HACKberry_R (Autodesk Fusion 360 archive; units mm, degrees)
design "SS12SDP2"
Autodesk Fusion 360 part; units mm, degrees
box "直方体プリミティブ1" add length 10.2 width 4 height 4.5 placed x (0, 0, 1) y (1, 0, 0) z (0, 1, 0) at (0, 0, 0) makes body 1
sketch "スケッチ2" plane through (0, 4.5, 0) normal (0, 1, 0) x (-1, 0, 0)
  line L0 (0, 10.2) -> (-4, 10.2)
  line L1 (-4, 10.2) -> (-4, 0)
  line L2 (-4, 0) -> (0, 0)
  line L3 (0, 0) -> (0, 10.2)
  line L4 (0, 0) -> (-4, 10.2) construction
  line L5 (0, 10.2) -> (-4, 0) construction
  line L6 (-2.6, 3.35) -> (-1.4, 3.35)
  line L7 (-1.4, 3.35) -> (-1.4, 6.85)
  line L8 (-1.4, 6.85) -> (-2.6, 6.85)
  line L9 (-2.6, 6.85) -> (-2.6, 3.35)
  line L10 (-2.6, 3.35) -> (-1.4, 6.85) construction
  line L11 (-1.4, 3.35) -> (-2.6, 6.85) construction
  point P0 (-2, 5.1)
  dimension "d6" = 1.2
  dimension "d7" = 3.5
  measures "d6" distance of L7.end L8.end
  measures "d7" distance of L6.end L7.end
extrude "押し出し1" cut sketch "スケッチ2" against normal blind 1 contours L6 L7 L8 L9 bodies 1
sketch "スケッチ3" plane through (0, 3.5, 0) normal (0, 1, 0) x (-1, 0, 0)
  line L0 (-2.6, 6.85) -> (-2.6, 3.35)
  line L1 (-2.6, 3.35) -> (-1.4, 3.35)
  line L2 (-1.4, 3.35) -> (-1.4, 6.85)
  line L3 (-1.4, 6.85) -> (-2.6, 6.85)
  line L4 (-1.4, 3.35) -> (-2.6, 3.35)
  line L5 (-2.6, 3.35) -> (-2.6, 5.1)
  line L6 (-2.6, 5.1) -> (-1.4, 5.1)
  line L7 (-1.4, 5.1) -> (-1.4, 3.35)
extrude "押し出し2" add sketch "スケッチ3" along normal blind 3 separate body contours L0 L1 L2 L4 L5 L6 L7 makes body 2
sketch "スケッチ4" plane through (0, 0, 0) normal (0, -1, 0) x (1, 0, 0)
  line L0 (4, 10.2) -> (0, 10.2)
  line L1 (0, 10.2) -> (0, 0)
  line L2 (0, 0) -> (4, 0)
  line L3 (4, 0) -> (4, 10.2)
  line L4 (2.2, 4.8) -> (1.8, 4.8)
  line L5 (1.8, 4.8) -> (1.8, 5.4)
  line L6 (1.8, 5.4) -> (2.2, 5.4)
  line L7 (2.2, 5.4) -> (2.2, 4.8)
  line L8 (2.2, 4.8) -> (1.8, 5.4) construction
  line L9 (1.8, 4.8) -> (2.2, 5.4) construction
  line L10 (1.4, 5.1) -> (2.6, 5.1)
  line L11 (1.8, 2.26) -> (1.8, 2.86)
  line L12 (2.2, 2.26) -> (1.8, 2.26)
  line L13 (1.8, 2.86) -> (2.2, 2.86)
  line L14 (2.2, 2.26) -> (1.8, 2.86) construction
  line L15 (1.8, 2.26) -> (2.2, 2.86) construction
  line L16 (2.2, 2.86) -> (2.2, 2.26)
  line L17 (1.8, 7.34) -> (1.8, 7.94)
  line L18 (2.2, 7.34) -> (1.8, 7.34)
  line L19 (1.8, 7.94) -> (2.2, 7.94)
  line L20 (2.2, 7.34) -> (1.8, 7.94) construction
  line L21 (1.8, 7.34) -> (2.2, 7.94) construction
  line L22 (2.2, 7.94) -> (2.2, 7.34)
  point P0 (2, 5.1)
  point P1 (2, 2.56)
  point P2 (2, 7.64)
  dimension "d12" = 0.4
  dimension "d13" = 0.6
  dimension "d16" = 0
  dimension "d17" = 2.54
  measures "d12" distance of L5.end L6.end
  measures "d13" distance of L4.end L5.end
extrude "押し出し3" add sketch "スケッチ4" along normal blind 3.4 separate body contours L4 L5 L7 L10 | L5 L6 L7 L10 | L11 L12 L13 L16 | L17 L18 L19 L22 makes body 3 at (1.8, -1.1333, 2.46) makes body 4 at (1.8, -1.1333, 7.54) makes body 5 at (2.2, -1.1333, 5.2)
chamfer "面取り1" distance 0.2 angle 45 8 edges at (2, 4.5, 10.2) (4, 2.25, 10.2) (4, 4.5, 5.1) (0, 4.5, 5.1) (0, 2.25, 10.2) (4, 2.25, 0) (2, 4.5, 0) (0, 2.25, 0) on bodies 1
sketch "スケッチ5" plane through (0, 0, 0) normal (-1, 0, 0) x (0, 0, 1)
  line L0 (0.2, 0) -> (10, 0)
  line L1 (0, 2.3446) -> (10.2, 2.3446)
  line L2 (10, 0) -> (10, 4.3)
  line L3 (10, 4.3) -> (0.2, 4.3)
  line L4 (0.2, 4.3) -> (0.2, 0)
split "分割1" by curves path "スケッチ5" along L1 bodies 1 makes body 6 at (1.3333, 0, 6.7333)
